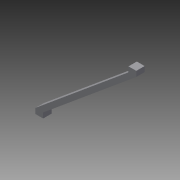
# Autodesk Inventor part: 1Pieceshortsupport_v1
Saved by Autodesk Inventor 2013 (Build 170138000, 138)
## iProperties
Created: 2013-01-19
Part Number: 1Pieceshortsupport_v1
Material: Generic
Document SubType Name: Modeling
Designer: motoennies
Density: 1 g/cm^3
Author: motoennies
Autodesk Inventor part; units mm, degrees
ref_plane "YZ Plane" through (0, 0, 0) normal (1, 0, 0) x (0, 1, 0)
ref_plane "XZ Plane" through (0, 0, 0) normal (0, 1, 0) x (-1, 0, 0)
ref_plane "XY Plane" through (0, 0, 0) normal (0, 0, 1) x (1, 0, 0)
sketch "Sketch1" plane through (0, 0, 0) normal (0, 0, 1) x (1, 0, 0)
  line L0 (0, 0) -> (9.525, 0)
  line L1 (9.525, 0) -> (9.525, 6.35)
  line L2 (0, 0) -> (0, 6.35)
  line L3 (113.3602, 100.5078) -> (113.3602, 106.8578)
  line L4 (113.3602, 106.8578) -> (122.8852, 106.8578)
  line L5 (122.8852, 106.8578) -> (122.8852, 100.5078)
  line L6 (9.525, 6.35) -> (122.8852, 100.5078)
  line L7 (0, 6.35) -> (113.3602, 100.5078)
  dimension "d0" = 9.525
  dimension "d1" = 6.35
  dimension "d2" = 6.35
  dimension "d3" = 9.525
  dimension "d4" = 103.8352
  dimension "d6" = 6.35
  dimension "d10" = 6.35
  dimension "d11" = 94.1578
  constraints: 16 end point, 3 parallel, 2 perpendicular, 1 horizontal
  measures "d0" distance of L0.start L0.end
  measures "d1" distance of L0.end L1.end
  measures "d2" distance of L3.start L3.end
  measures "d3" distance of L3.end L4.end
  measures "d4" distance between parallel lines of L3 L1
  measures "d6" distance of L4.end L5.end
  measures "d10" distance of L0.start L2.end
  measures "d11" vertical distance of L5.end L1.end
extrude "Extrusion1" add sketch "Sketch1" along normal blind 10.16
body "Solid1"
